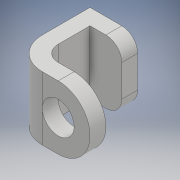
# Autodesk Inventor part: 18
Saved by Autodesk Inventor 2017 (Build 210142000, 142)
## iProperties
Part Number: 18
Material: 一般
Document SubType Name: Modeling
Designer: Brian
Density: 1 g/cm^3
Appearance: 預設
Author: Brian
Autodesk Inventor part; units mm, degrees
ref_plane "YZ Plane" through (0, 0, 0) normal (1, 0, 0) x (0, 1, 0)
ref_plane "XZ Plane" through (0, 0, 0) normal (0, 1, 0) x (-1, 0, 0)
ref_plane "XY Plane" through (0, 0, 0) normal (0, 0, 1) x (1, 0, 0)
sketch "草圖1" plane through (0, 0, 0) normal (0, 0, 1) x (1, 0, 0)
  line L0 (0, 0) -> (10, 0)
  line L1 (10, 0) -> (10, 50)
  line L2 (10, 50) -> (0, 50)
  line L3 (0, 50) -> (0, 0)
  line L4 (10, 0) -> (50, 0)
  line L5 (50, 0) -> (50, 10)
  line L6 (50, 10) -> (10, 10)
  line L7 (10, 10) -> (10, 0)
  line L8 (10, 50) -> (30, 50)
  line L9 (30, 50) -> (30, 40)
  line L10 (30, 40) -> (10, 40)
  line L11 (10, 40) -> (10, 50)
  dimension "d0" = 10
  dimension "d1" = 10
  dimension "d2" = 20
  dimension "d3" = 40
  dimension "d4" = 10
  dimension "d5" = 50
  constraints: 24 end point, 6 parallel, 3 horizontal, 3 perpendicular
  measures "d0" distance of L8.end L9.end
  measures "d1" distance of L1.end L2.end
  measures "d2" distance of L1.end L8.end
  measures "d3" distance of L5.end L6.end
  measures "d4" distance of L4.end L5.end
  measures "d5" distance of L0.end L1.end
extrude "擠出1" add sketch "草圖1" along normal blind 40
fillet "圓角1" radius 10 1 edges at (10, 10, 20)
fillet "圓角2" radius 10 2 edges at (30, 45, 40) (30, 45, 0)
fillet "圓角3" radius 20 3 edges at (0, 0, 20) (50, 5, 40) (50, 5, 0)
sketch "草圖2" plane through (20, 10, 40) normal (0, 1, 0) x (1, 0, 0)
  arc A0 (10, 0) -> (10, 40) centre (10, 20) ccw projected
  circle A1 centre (10, 20) radius 10
  point P0 (-20, 40)
  dimension "d11" = 20
  constraints: 1 centre point, 1 coincident
  measures "d11" diameter of A1
extrude "擠出2" cut sketch "草圖2" against normal blind 40
